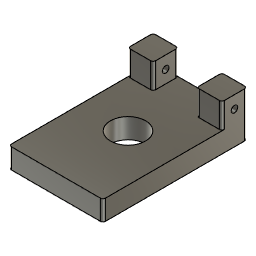
Single_Protected_Base (Autodesk Fusion 360 design; units mm, degrees)
Autodesk Fusion 360 part; units mm, degrees
sketch "Sketch1" plane through (0, 0, 0) normal (0, 0, 1) x (1, 0, 0)
  line L0 (0.5, 0) -> (18.2, 0)
  line L1 (18.7, 0.5) -> (18.7, 28.2)
  line L2 (18.2, 28.7) -> (0.5, 28.7)
  line L3 (0, 28.2) -> (0, 0.5)
  line L4 (18.7, 28.7) -> (0, 0) construction
  line L5 (0, 28.7) -> (18.7, 0) construction
  arc A0 (0.5, 28.7) -> (0, 28.2) centre (0.5, 28.2) ccw
  arc A1 (18.7, 28.2) -> (18.2, 28.7) centre (18.2, 28.2) ccw
  arc A2 (18.2, 0) -> (18.7, 0.5) centre (18.2, 0.5) ccw
  arc A3 (0, 0.5) -> (0.5, 0) centre (0.5, 0.5) ccw
  circle A4 centre (9.35, 14.35) radius 3.5
  dimension "d1" = 18.7
  dimension "d2" = 28.7
  dimension "d3" = 0.5
  dimension "d4" = 0.5
  dimension "d5" = 0.5
  dimension "d6" = 0.5
  dimension "d7" = 7
  constraint horizontal L0
  constraint vertical L1
  constraint horizontal L2
  constraint vertical L3
  constraint coincident L4.end origin
  constraint coincident L5.start L2
  constraint coincident L5.start L3
  constraint tangent L2 A0
  constraint tangent L3 A0
  constraint coincident L4.start L1
  constraint coincident L4.start L2
  constraint tangent L1 A1
  constraint tangent L2 A1
  constraint coincident L5.end L0
  constraint coincident L5.end L1
  constraint tangent L0 A2
  constraint tangent L1 A2
  constraint coincident L4.end L0
  constraint coincident L4.end L3
  constraint tangent L0 A3
  constraint tangent L3 A3
  constraint midpoint L4 A4.centre
  measures "d1" distance of L4.end L5.end
  measures "d2" distance of L4.end L5.start
  measures "d3" radius of A0
  measures "d4" radius of A1
  measures "d5" radius of A2
  measures "d6" radius of A3
  measures "d7" diameter of A4
extrude "Extrude1" add sketch "Sketch1" along normal blind 4
sketch "Sketch2" plane through (0, 0, 4) normal (0, 0, 1) x (-1, 0, 0)
  circle A0 centre (-9.35, -14.35) radius 3.5
  arc A1 (0, -0.5) -> (-0.5, 0) centre (-0.5, -0.5) ccw
  line L0 (-0.5, 0) -> (-18.2, 0)
  arc A2 (-18.2, 0) -> (-18.7, -0.5) centre (-18.2, -0.5) ccw
  line L1 (-18.7, -0.5) -> (-18.7, -28.2)
  arc A3 (-18.7, -28.2) -> (-18.2, -28.7) centre (-18.2, -28.2) ccw
  line L2 (-18.2, -28.7) -> (-0.5, -28.7)
  arc A4 (-0.5, -28.7) -> (0, -28.2) centre (-0.5, -28.2) ccw
  line L3 (0, -28.2) -> (0, -0.5)
  line L4 (-9.35, -23.7) -> (-18.2, -23.7) construction
  line L5 (-9.35, -23.7) -> (0, -23.7) construction
  line L6 (-18.7, -23.7) -> (-14.2, -23.7)
  line L7 (-0.5, -23.7) -> (-4.5, -23.7)
  line L8 (-5, -24.2) -> (-5, -28.2)
  line L9 (-13.7, -24.2) -> (-13.7, -28.2)
  line L10 (-14.2, -28.7) -> (-18.2, -28.7)
  line L11 (-18.7, -28.2) -> (-18.7, -24.2)
  line L12 (-4.5, -28.7) -> (-0.5, -28.7)
  line L13 (0, -28.2) -> (0, -24.2)
  arc A5 (-0.5, -28.7) -> (0, -28.2) centre (-0.5, -28.2) ccw
  arc A6 (-18.7, -28.2) -> (-18.2, -28.7) centre (-18.2, -28.2) ccw
  arc A7 (-4.5, -23.7) -> (-5, -24.2) centre (-4.5, -24.2) ccw
  arc A8 (0, -24.2) -> (-0.5, -23.7) centre (-0.5, -24.2) ccw
  arc A9 (-5, -28.2) -> (-4.5, -28.7) centre (-4.5, -28.2) ccw
  arc A10 (-14.2, -28.7) -> (-13.7, -28.2) centre (-14.2, -28.2) ccw
  arc A11 (-13.7, -24.2) -> (-14.2, -23.7) centre (-14.2, -24.2) ccw
  arc A12 (-18.2, -23.7) -> (-18.7, -24.2) centre (-18.2, -24.2) ccw
  point P0 (-5, -28.7)
  point P1 (-13.7, -28.7)
  point P2 (-18.7, -28.7)
  point P3 (0, -28.7)
  dimension "d12" = 5
  dimension "d13" = 5
  dimension "d14" = 0.5
  dimension "d15" = 0.5
  dimension "d16" = 0.5
  dimension "d17" = 0.5
  dimension "d18" = 0.5
  dimension "d19" = 0.5
  dimension "d20" = 0.5
  dimension "d21" = 0.5
  constraint coincident L1 L6.start
  constraint perpendicular L1 L4
  constraint coincident L3 L5.end
  constraint perpendicular L3 L5
  constraint perpendicular L1 L6
  constraint coincident L2 P0
  constraint perpendicular L2 L8
  constraint perpendicular L4 L9
  constraint perpendicular L9 L10
  constraint perpendicular L10 L11
  constraint perpendicular L8 L12
  constraint coincident P3 L12
  constraint coincident P3 L13
  constraint tangent L12 A5
  constraint tangent L13 A5
  constraint coincident P2 L10
  constraint coincident P2 L11
  constraint tangent L10 A6
  constraint tangent L11 A6
  constraint tangent L7 A7
  constraint tangent L8 A7
  constraint coincident L5.end L7
  constraint coincident L5.end L13
  constraint tangent L7 A8
  constraint tangent L13 A8
  constraint coincident P0 L8
  constraint coincident P0 L12
  constraint tangent L8 A9
  constraint tangent L12 A9
  constraint coincident P1 L9
  constraint coincident P1 L10
  constraint tangent L9 A10
  constraint tangent L10 A10
  constraint tangent L6 A11
  constraint tangent L9 A11
  constraint coincident L6.start L4
  constraint coincident L6.start L11
  constraint tangent L4 A12
  constraint tangent L11 A12
  measures "d12" distance of P1 P2
  measures "d13" distance of P0 P3
  measures "d14" radius of A5
  measures "d15" radius of A6
  measures "d16" radius of A7
  measures "d17" radius of A8
  measures "d18" radius of A9
  measures "d19" radius of A10
  measures "d20" radius of A11
  measures "d21" radius of A12
extrude "Extrude2" add sketch "Sketch2" along normal blind 5 contours L2 A4 L3 L7 L8 L12 L13 A5 A7 A8 A9 | L1 A3 L2 L6 L9 L10 L11 A6 A10 A11 A12
sketch "Sketch3" plane through (18.7, 0, 0) normal (1, 0, 0) x (0, 1, 0)
  line L0 (0.5, 0) -> (28.2, 0)
  line L1 (28.2, 0) -> (28.2, 9)
  line L2 (28.2, 9) -> (24.2, 9)
  line L3 (24.2, 9) -> (24.2, 4)
  line L4 (24.2, 4) -> (0.5, 4)
  line L5 (0.5, 4) -> (0.5, 0)
  line L6 (24.2, 9) -> (24.2, 4) construction
  line L7 (24.2, 4) -> (28.2, 4) construction
  line L8 (24.2, 9) -> (28.2, 4) construction
  line L9 (24.2, 4) -> (28.2, 9) construction
  circle A0 centre (26.2, 6.5) radius 0.65
  dimension "d24" = 1.3
  constraint coincident L2.end L3.start
  constraint coincident L3.end L4.start
  constraint coincident L1 L7.end
  constraint perpendicular L1 L7
  constraint coincident L1.end L2.start
  constraint midpoint L9 A0.centre
  measures "d24" diameter of A0
extrude "Extrude3" cut sketch "Sketch3" against normal blind 20 contours A0
